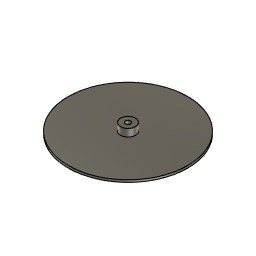
lid v2 (Autodesk Fusion 360 design; units mm, degrees)
Autodesk Fusion 360 part; units mm, degrees
sketch "スケッチ1" plane through (0, 0, 0) normal (0, 0, 1) x (1, 0, 0)
  circle A0 centre (0, 0) radius 80
  circle A1 centre (0, 0) radius 3.5
  dimension "d1" = 160
  dimension "d7" = 7
  constraint coincident A0.centre A1.centre
  constraint concentric A0 A1
  measures "d1" diameter of A0
  measures "d7" diameter of A1
extrude "押し出し1" add sketch "スケッチ1" along normal blind 3 contours A0 | A1
sketch "スケッチ2" plane through (0, 0, 3) normal (0, 0, 1) x (-1, 0, 0)
  circle A0 centre (0, 0) radius 80
  circle A1 centre (0, 0) radius 10
  dimension "d4" = 20
  constraint concentric A0 A1
  measures "d4" diameter of A1
extrude "押し出し2" add sketch "スケッチ2" along normal blind 10 contours A1
extrude "押し出し3" cut sketch "スケッチ1" along normal blind 13 contours A1
